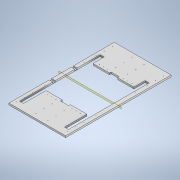
# Autodesk Inventor part: top_part
Saved by Autodesk Inventor 2020 (Build 240168000, 168)
## iProperties
Created: 2019-12-27
Part Number: top_part
Material: Générique
Document SubType Name: Modeling
Designer: damien
Density: 1 g/cm^3
Appearance: Par défaut
Author: damien
Autodesk Inventor part; units mm, degrees
ref_plane "YZ Plane" through (0, 0, 0) normal (1, 0, 0) x (0, 1, 0)
ref_plane "XZ Plane" through (0, 0, 0) normal (0, 1, 0) x (-1, 0, 0)
ref_plane "XY Plane" through (0, 0, 0) normal (0, 0, 1) x (1, 0, 0)
sketch "Esquisse1" plane through (0, 0, 0) normal (0, 1, 0) x (-1, 0, 0)
  line L0 (-350, -650) -> (350, -650)
  line L1 (350, -650) -> (350, 650)
  line L2 (350, 650) -> (-350, 650)
  line L3 (-350, 650) -> (-350, -650)
  line L4 (-350, -650) -> (350, 650) construction
  line L5 (350, -650) -> (-350, 650) construction
  point P0 (0, 0)
  dimension "d0" = 1300
  dimension "d1" = 700
  constraints: 12 end point, 2 midpoint, 2 parallel, 1 horizontal, 1 perpendicular
  measures "d0" distance of L0.end L1.end
  measures "d1" distance of L1.end L2.end
extrude "Extrusion1" add sketch "Esquisse1" along normal blind 20.7
sketch "Esquisse2" plane through (0, 20.7, 0) normal (0, 1, 0) x (1, 0, 0)
  line L0 (-305, -565.5) -> (-305, 429.5)
  line L1 (-305, 429.5) -> (-255, 429.5)
  line L2 (-255, 429.5) -> (-255, 292.5)
  line L3 (-255, 292.5) -> (250, 292.5)
  line L4 (250, 292.5) -> (250, 429.5)
  line L5 (250, 429.5) -> (300, 429.5)
  line L6 (300, 429.5) -> (300, -565.5)
  line L7 (300, -565.5) -> (250, -565.5)
  line L8 (250, -565.5) -> (250, -287.5)
  line L9 (250, -287.5) -> (-255, -287.5)
  line L10 (-255, -287.5) -> (-255, -565.5)
  line L11 (-255, -565.5) -> (-305, -565.5)
  line L12 (350, -650) -> (350, 650) projected
  line L13 (350, 0) -> (300, -68) construction
  line L14 (-350, 650) -> (-350, -650) projected
  line L15 (-350, -650) -> (350, -650) projected
  point P0 (0, 0)
  dimension "d4" = 995
  dimension "d5" = 50
  dimension "d6" = 605
  dimension "d7" = 580
  dimension "d8" = 137
  dimension "d9" = 50
  dimension "d10" = 84.5
  constraints: 26 end point, 7 perpendicular, 6 point on line, 2 equal length, 2 midpoint, 2 vertical
  measures "d4" distance of L5.end L6.end
  measures "d5" distance of L6.end L7.end
  measures "d6" distance between parallel lines of L0 L6
  measures "d7" distance between parallel lines of L3 L9
  measures "d8" distance of L3.end L4.end
  measures "d9" distance between parallel lines of L12 L6
  measures "d10" distance between parallel lines of L15 L11
extrude "Extrusion2" cut sketch "Esquisse2" against normal blind 21.1
sketch "Esquisse3" plane through (-350, 0, 650) normal (1, 0, 0) x (0, 0, -1)
  line L0 (84.5, 20.7) -> (1079.5, 20.7) projected
  line L1 (495, 20.7) -> (525, 20.7)
  line L2 (525, 20.7) -> (525, 5.7)
  line L3 (525, 5.7) -> (495, 5.7)
  line L4 (495, 5.7) -> (495, 20.7)
  line L5 (0, 0) -> (0, 20.7) projected
  line L6 (765, 20.7) -> (795, 20.7)
  line L7 (795, 20.7) -> (795, 5.7)
  line L8 (795, 5.7) -> (765, 5.7)
  line L9 (765, 5.7) -> (765, 20.7)
  point P0 (650, 0)
  dimension "d13" = 495
  dimension "d14" = 30
  dimension "d15" = 15
  dimension "d16" = 240
  dimension "d17" = 30
  constraints: 16 end point, 4 parallel, 2 horizontal, 2 perpendicular, 2 point on line, 1 collinear
  measures "d13" distance from line of L5 L1.start
  measures "d14" distance of L2.end L3.end
  measures "d15" distance of L1.end L2.end
  measures "d16" distance between parallel lines of L9 L2
  measures "d17" distance of L7.end L8.end
extrude "Extrusion3" cut sketch "Esquisse3" along normal blind 100
sketch "Esquisse4" plane through (0, 20.7, 0) normal (0, 1, 0) x (1, 0, 0)
  line L0 (250, 292.5) -> (-255, 292.5) projected
  line L1 (-52.5, 292.5) -> (47.5, 292.5)
  line L2 (47.5, 292.5) -> (47.5, 312.5)
  line L3 (47.5, 312.5) -> (-52.5, 312.5)
  line L4 (-52.5, 312.5) -> (-52.5, 292.5)
  line L5 (-255, -287.5) -> (250, -287.5) projected
  line L6 (-52.5, -287.5) -> (47.5, -287.5)
  line L7 (47.5, -287.5) -> (47.5, -310.5)
  line L8 (47.5, -310.5) -> (-52.5, -310.5)
  line L9 (-52.5, -310.5) -> (-52.5, -287.5)
  line L10 (-255, 429.5) -> (-255, 292.5) projected
  line L11 (250, 292.5) -> (250, 429.5) projected
  point P0 (0, 0)
  point P1 (47.5, -287.5)
  dimension "d20" = 23
  dimension "d21" = 100
  dimension "d22" = 202.5
  dimension "d23" = 202.5
  dimension "d50" = 20
  constraints: 16 end point, 4 parallel, 4 point on line, 2 horizontal, 2 perpendicular
  measures "d20" distance of L6.end L7.end
  measures "d21" distance of L2.end L3.end
  measures "d22" distance between parallel lines of L10 L4
  measures "d23" distance between parallel lines of L11 L2
  measures "d50" distance of L1.end L2.end
extrude "Extrusion4" cut sketch "Esquisse4" against normal blind 100
fillet "Congé1" radius 2 8 edges at (47.5, 10.35, -312.5) (47.5, 10.35, -292.5) (-52.5, 10.35, -312.5) (-52.5, 10.35, -292.5) (-52.5, 10.35, 287.5) (-52.5, 10.35, 310.5) (47.5, 10.35, 310.5) (47.5, 10.35, 287.5)
sketch "Esquisse5" plane through (0, 20.7, 0) normal (0, 1, 0) x (1, 0, 0)
  circle A0 centre (-74, 492.5) radius 2.25
  circle A1 centre (-74, 392.5) radius 2.25
  line L0 (-350, 650) -> (-350, 145) projected
  circle A2 centre (73, 392.5) radius 2.25
  line L1 (350, -650) -> (350, 650) projected
  circle A3 centre (73, 492.5) radius 2.25
  circle A4 centre (-74, 592.5) radius 2.25
  circle A5 centre (73, 592.5) radius 2.25
  line L2 (-255, 292.5) -> (-54.5, 292.5) projected
  circle A6 centre (316, 592.5) radius 2.25
  circle A7 centre (316, 492.5) radius 2.25
  circle A8 centre (316, 392.5) radius 2.25
  circle A9 centre (-318, 392.5) radius 2.25
  circle A10 centre (-318, 492.5) radius 2.25
  circle A11 centre (-318, 592.5) radius 2.25
  circle A12 centre (-318, 242.5) radius 2.25
  circle A13 centre (316, 242.5) radius 2.25
  point P0 (0, 0)
  dimension "d27" = 276
  dimension "d28" = 277
  dimension "d29" = 100
  dimension "d30" = 100
  dimension "d31" = 4.5
  dimension "d32" = 100
  dimension "d35" = 34
  dimension "d36" = 32
  dimension "d51" = 150
  constraints: 14 centre point, 13 equal radius, 10 horizontal alignment, 10 vertical alignment
  measures "d27" distance from line of L0 A1.centre
  measures "d28" distance from line of L1 A2.centre
  measures "d29" distance of A0.centre A1.centre
  measures "d30" distance of A0.centre A4.centre
  measures "d31" diameter of A2
  measures "d32" distance from line of A1.centre L2
  measures "d35" distance from line of L1 A7.centre
  measures "d36" distance from line of L0 A9.centre
  measures "d51" distance of A12.centre A9.centre
extrude "Extrusion5" cut sketch "Esquisse5" against normal blind 100
mirror "Symétrie1" about plane through (0, 0, 0) normal (0, 0, 1) of "Extrusion5"
sketch "Esquisse6" plane through (0, 20.7, 0) normal (0, 1, 0) x (1, 0, 0)
  circle A0 centre (-202.5, -319.5) radius 2.25
  line L0 (-255, -565.5) -> (-255, -287.5) projected
  line L1 (-255, -319.5) -> (250, -319.5) construction
  line L2 (250, -565.5) -> (250, -287.5) projected
  line L3 (45.5, -310.5) -> (-50.5, -310.5) projected
  circle A1 centre (-152.5, -319.5) radius 2.25
  circle A2 centre (-102.5, -319.5) radius 2.25
  line L4 (-50.5, -310.5) -> (45.5, -310.5) projected
  line L5 (-2.5, -310.5) -> (-2.5, -650) construction
  line L6 (-350, -650) -> (350, -650) projected
  circle A3 centre (197.5, -319.5) radius 2.25
  circle A4 centre (147.5, -319.5) radius 2.25
  circle A5 centre (97.5, -319.5) radius 2.25
  point P0 (0, 0)
  dimension "d37" = 4.5
  dimension "d38" = 9
  dimension "d39" = 52.5
  dimension "d42" = 50
  constraints: 6 centre point, 4 end point, 4 point on line, 3 symmetric about line, 2 horizontal, 2 midpoint, 1 vertical, 7 other
  measures "d37" diameter of A0
  measures "d38" distance between parallel lines of L1 L3
  measures "d39" distance from line of L0 A0.centre
  measures "d42" distance of A0.centre A1.centre
extrude "Extrusion6" cut sketch "Esquisse6" against normal blind 100
mirror "Symétrie3" about plane through (0, 0, 0) normal (0, 0, 1) of "Extrusion6"
ref_plane "Plan de construction1" through (0, 0, 0) normal (0, 0, 1) x (1, 0, 0)
